Autodesk Fusion 360 part; units mm, degrees
(part 3 of 3)
sketch "Battery (placeholder 7.0 x 3.5 x 2.5) sketch" plane through (0, 0, 0) normal (0, 0, 1) x (1, 0, 0) in component "Battery"
  line L0 (7.5706, 20.1882) -> (76.5071, 32.3436)
  line L1 (76.5071, 32.3436) -> (70.4294, 66.8118)
  line L2 (70.4294, 66.8118) -> (1.4929, 54.6564)
  line L3 (1.4929, 54.6564) -> (7.5706, 20.1882)
extrude "Battery (placeholder 7.0 x 3.5 x 2.5)" add sketch "Battery (placeholder 7.0 x 3.5 x 2.5) sketch" along normal blind 25 from surface at 51 separate body makes body 94 in component "Battery"
sketch "Floor sensor FP (black, blue, red) sketch" plane through (0, 0, 0) normal (0, 0, 1) x (1, 0, 0) in component "Floor port FP"
  line L0 (67, 24) -> (83, 24)
  line L1 (83, 24) -> (83, 40)
  line L2 (83, 40) -> (67, 40)
  line L3 (67, 40) -> (67, 24)
extrude "Floor sensor FP (black, blue, red)" add sketch "Floor sensor FP (black, blue, red) sketch" along normal blind 14 from surface at 28 separate body makes body 95 in component "Floor port FP"
sketch "Silver module SM (straight + 20 deg tilted pair) sketch" plane through (0, 0, 0) normal (0, 0, 1) x (1, 0, 0) in component "Silver module SM"
  line L0 (65, -38) -> (85, -38)
  line L1 (85, -38) -> (85, -16)
  line L2 (85, -16) -> (65, -16)
  line L3 (65, -16) -> (65, -38)
extrude "Silver module SM (straight + 20 deg tilted pair)" add sketch "Silver module SM (straight + 20 deg tilted pair) sketch" along normal blind 14 from surface at 28 separate body makes body 96 in component "Silver module SM"
sketch "USB-C J12 sketch" plane through (0, 0, 0) normal (0, 0, 1) x (1, 0, 0) in component "Arduino GIGA R1"
  line L0 (72.96, -31.93) -> (76.96, -31.93)
  line L1 (76.96, -31.93) -> (76.96, -22.93)
  line L2 (76.96, -22.93) -> (72.96, -22.93)
  line L3 (72.96, -22.93) -> (72.96, -31.93)
extrude "USB-C J12" add sketch "USB-C J12 sketch" along normal blind 3.5 from surface at 63.1 separate body makes body 97 in component "Arduino GIGA R1"
sketch "Wi-Fi antenna sketch" plane through (0, 0, 0) normal (0, 0, 1) x (1, 0, 0) in component "Wi-Fi antenna"
  line L0 (101.5046, -13.8862) -> (102.0018, -13.9384)
  line L1 (102.0018, -13.9384) -> (102.6708, -7.5735)
  line L2 (102.6708, -7.5735) -> (102.1735, -7.5212)
  line L3 (102.1735, -7.5212) -> (101.5046, -13.8862)
extrude "Wi-Fi antenna" add sketch "Wi-Fi antenna sketch" along normal blind 15.4 from surface at 55 separate body makes body 98 in component "Wi-Fi antenna"
sketch "Body sketch" plane through (0, 0, 0) normal (0, 0, 1) x (1, 0, 0) in component "Stepper bay 28BYJ-48"
  circle A0 centre (-14.8577, 6.1284) radius 14
extrude "Body" add sketch "Body sketch" along normal blind 19 from surface at 68 separate body makes body 99 in component "Stepper bay 28BYJ-48"
sketch "Ear sketch" plane through (0, 0, 0) normal (0, 0, 1) x (1, 0, 0) in component "Stepper bay 28BYJ-48"
  line L0 (-3.4154, 1.0961) -> (0.7978, -2.4393)
  arc A0 (-3.7017, -7.8016) -> (0.7978, -2.4393) centre (-1.4519, -5.1204) ccw
  line L1 (-3.7017, -7.8016) -> (-7.9149, -4.2663)
  arc A1 (-3.4154, 1.0961) -> (-7.9149, -4.2663) centre (-5.6652, -1.5851) ccw
extrude "Ear" add sketch "Ear sketch" along normal blind 7 from surface at 80 bodies 99 in component "Stepper bay 28BYJ-48"
sketch "Ear sketch (1)" plane through (0, 0, 0) normal (0, 0, 1) x (1, 0, 0) in component "Stepper bay 28BYJ-48"
  line L0 (-26.3, 11.1607) -> (-30.5132, 14.696)
  arc A0 (-26.0137, 20.0583) -> (-30.5132, 14.696) centre (-28.2635, 17.3771) ccw
  line L1 (-26.0137, 20.0583) -> (-21.8005, 16.523)
  arc A1 (-26.3, 11.1607) -> (-21.8005, 16.523) centre (-24.0502, 13.8418) ccw
extrude "Ear (1)" add sketch "Ear sketch (1)" along normal blind 7 from surface at 80 bodies 99 in component "Stepper bay 28BYJ-48"
sketch "Wire block sketch" plane through (0, 0, 0) normal (0, 0, 1) x (1, 0, 0) in component "Stepper bay 28BYJ-48"
  line L0 (-9.5224, 23.8435) -> (-12.7364, 20.0132)
  line L1 (-12.7364, 20.0132) -> (-1.5521, 10.6285)
  line L2 (-1.5521, 10.6285) -> (1.6618, 14.4588)
  line L3 (1.6618, 14.4588) -> (-9.5224, 23.8435)
extrude "Wire block" add sketch "Wire block sketch" along normal blind 19 from surface at 68 bodies 99 in component "Stepper bay 28BYJ-48"
component "Tub" placed x (1, 0, 0) y (0, 1, 0) z (0, 0, 1) at (0, 0, 0)
component "Wheel L" placed x (1, 0, 0) y (0, 1, 0) z (0, 0, 1) at (0, 0, 0)
component "Motor L" placed x (1, 0, 0) y (0, 1, 0) z (0, 0, 1) at (0, 0, 0)
component "Wheel R" placed x (1, 0, 0) y (0, 1, 0) z (0, 0, 1) at (0, 0, 0)
component "Motor R" placed x (1, 0, 0) y (0, 1, 0) z (0, 0, 1) at (0, 0, 0)
component "Face plate L" placed x (1, 0, 0) y (0, 1, 0) z (0, 0, 1) at (0, 0, 0)
component "Face plate R" placed x (1, 0, 0) y (0, 1, 0) z (0, 0, 1) at (0, 0, 0)
component "Omni wheel" placed x (1, 0, 0) y (0, 1, 0) z (0, 0, 1) at (0, 0, 0)
component "Omni arm" placed x (1, 0, 0) y (0, 1, 0) z (0, 0, 1) at (0, 0, 0)
component "Omni pins" placed x (1, 0, 0) y (0, 1, 0) z (0, 0, 1) at (0, 0, 0)
component "Rear nub" placed x (1, 0, 0) y (0, 1, 0) z (0, 0, 1) at (0, 0, 0)
component "Bumper L" placed x (1, 0, 0) y (0, 1, 0) z (0, 0, 1) at (0, 0, 0)
component "Bumper switch L" placed x (1, 0, 0) y (0, 1, 0) z (0, 0, 1) at (0, 0, 0)
component "Bumper R" placed x (1, 0, 0) y (0, 1, 0) z (0, 0, 1) at (0, 0, 0)
component "Bumper switch R" placed x (1, 0, 0) y (0, 1, 0) z (0, 0, 1) at (0, 0, 0)
component "Upper frame" placed x (1, 0, 0) y (0, 1, 0) z (0, 0, 1) at (0, 0, 0)
component "ToF F" placed x (1, 0, 0) y (0, 1, 0) z (0, 0, 1) at (0, 0, 0)
component "ToF FL" placed x (1, 0, 0) y (0, 1, 0) z (0, 0, 1) at (0, 0, 0)
component "ToF FR" placed x (1, 0, 0) y (0, 1, 0) z (0, 0, 1) at (0, 0, 0)
component "ToF SFL" placed x (1, 0, 0) y (0, 1, 0) z (0, 0, 1) at (0, 0, 0)
component "ToF SFR" placed x (1, 0, 0) y (0, 1, 0) z (0, 0, 1) at (0, 0, 0)
component "ToF SRL" placed x (1, 0, 0) y (0, 1, 0) z (0, 0, 1) at (0, 0, 0)
component "ToF SRR" placed x (1, 0, 0) y (0, 1, 0) z (0, 0, 1) at (0, 0, 0)
component "ToF RL" placed x (1, 0, 0) y (0, 1, 0) z (0, 0, 1) at (0, 0, 0)
component "ToF RR" placed x (1, 0, 0) y (0, 1, 0) z (0, 0, 1) at (0, 0, 0)
component "Camera L" placed x (1, 0, 0) y (0, 0.34202, 0.939693) z (0, -0.939693, 0.34202) at (3.0712, 87.9464, 93)
component "Camera R" placed x (-1, 0, 0) y (0, -0.34202, 0.939693) z (0, 0.939693, 0.34202) at (3.0712, -87.9464, 93)
component "Lid" placed x (1, 0, 0) y (0, 1, 0) z (0, 0, 1) at (0, 0, 0)
component "Handle bar" placed x (1, 0, 0) y (0, 1, 0) z (0, 0, 1) at (0, 0, 0)
component "Victim LED" placed x (1, 0, 0) y (0, 1, 0) z (0, 0, 1) at (0, 0, 0)
component "Start button" placed x (1, 0, 0) y (0, 1, 0) z (0, 0, 1) at (0, 0, 0)
component "Power switch" placed x (1, 0, 0) y (0, 1, 0) z (0, 0, 1) at (0, 0, 0)
component "Status LED 1" placed x (1, 0, 0) y (0, 1, 0) z (0, 0, 1) at (0, 0, 0)
component "Status LED 2" placed x (1, 0, 0) y (0, 1, 0) z (0, 0, 1) at (0, 0, 0)
component "USB-C service socket" placed x (1, 0, 0) y (0, 1, 0) z (0, 0, 1) at (0, 0, 0)
component "Dropper floor" placed x (1, 0, 0) y (0, 1, 0) z (0, 0, 1) at (0, 0, 0)
component "Dropper plate" placed x (1, 0, 0) y (0, 1, 0) z (0, 0, 1) at (0, 0, 0)
component "N20 motor" placed x (1, 0, 0) y (0, 1, 0) z (0, 0, 1) at (0, 0, 0)
component "N20 face plate" placed x (1, 0, 0) y (0, 1, 0) z (0, 0, 1) at (0, 0, 0)
component "Kits" placed x (1, 0, 0) y (0, 1, 0) z (0, 0, 1) at (0, 0, 0)
component "Hopper B left" placed x (1, 0, 0) y (0, 1, 0) z (0, 0, 1) at (0, 0, 0)
component "Chute B left" placed x (1, 0, 0) y (0, 1, 0) z (0, 0, 1) at (0, 0, 0)
component "Hopper A right" placed x (1, 0, 0) y (0, 1, 0) z (0, 0, 1) at (0, 0, 0)
component "Chute A right" placed x (1, 0, 0) y (0, 1, 0) z (0, 0, 1) at (0, 0, 0)
component "GIGA posts" placed x (1, 0, 0) y (0, 1, 0) z (0, 0, 1) at (0, 0, 0)
component "Arduino GIGA R1" placed x (1, 0, 0) y (0, 1, 0) z (0, 0, 1) at (0, 0, 0)
component "Main PCB" placed x (1, 0, 0) y (0, 1, 0) z (0, 0, 1) at (0, 0, 0)
component "Battery" placed x (1, 0, 0) y (0, 1, 0) z (0, 0, 1) at (0, 0, 0)
component "Floor port FP" placed x (1, 0, 0) y (0, 1, 0) z (0, 0, 1) at (0, 0, 0)
component "Silver module SM" placed x (1, 0, 0) y (0, 1, 0) z (0, 0, 1) at (0, 0, 0)
component "Wi-Fi antenna" placed x (1, 0, 0) y (0, 1, 0) z (0, 0, 1) at (0, 0, 0)
component "Stepper bay 28BYJ-48" placed x (1, 0, 0) y (0, 1, 0) z (0, 0, 1) at (0, 0, 0)
named bodies: "Tub shell", "Chute hole tool B left", "Chute hole tool A right", "Cradle prong front L", "Cradle prong rear L", "Cradle prong front R", "Cradle prong rear R", "Wheel L", "Encoder L", "Gearmotor L", "Motor shaft L", "Wheel R", "Encoder R", "Gearmotor R", "Motor shaft R", "Face plate L", "Face plate R", "Omni wheel", "Arm plate", "Pivot pin", "Axle pin", "Rear nub", "Bumper plate L", "Microswitch L", "Bumper plate R", "Microswitch R", "Frame ring", "VL53L0X module F", "VL53L0X chip F", "VL53L0X module FL", "VL53L0X chip FL", "VL53L0X module FR", "VL53L0X chip FR", "VL53L0X module SFL", "VL53L0X chip SFL", "VL53L0X module SFR", "VL53L0X chip SFR", "VL53L0X module SRL", "VL53L0X chip SRL", "VL53L0X module SRR", "VL53L0X chip SRR", "VL53L0X module RL", "VL53L0X chip RL", "VL53L0X module RR", "VL53L0X chip RR", "Lens block L", "OpenMV H7 Plus board L", "Lens block R", "OpenMV H7 Plus board R", "Lid plate", "Hook bump +71", "Hook bump +114", "Hook bump -71", "Hook bump -114", "Handle bar", "Victim LED", "Start button", "Power switch", "Status LED 1", "Status LED 2", "USB-C service socket", "Dropper floor", "Dropper plate", "N20 gearmotor with encoder", "N20 shaft", "N20 face plate", "Kit 1", "Kit 2", "Kit 3", "Kit 4", "Kit 5", "Kit 6", "Kit 7", "Kit 8", "Hopper", "Socket tool", "Channel", "Channel void", "Trim", "GIGA post H1", "GIGA post H2", "GIGA post H3", "GIGA post H4", "GIGA board", "Header strip +y", "Header strip -y", "Main PCB shield (placeholder)", "PCB component envelope (placeholder)", "Battery (placeholder 7.0 x 3.5 x 2.5)", "Floor sensor FP (black, blue, red)", "Silver module SM (straight + 20 deg tilted pair)", "USB-C J12", "Wi-Fi antenna", "Body"
